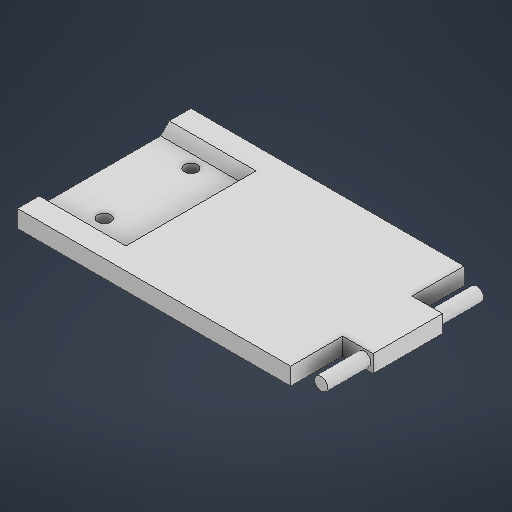
# Autodesk Inventor part: upper
Saved by Autodesk Inventor 2026.1 (Build 301233020, 233B)
## iProperties
Created: 2026-08-26
Part Number: upper
Material: Generic
Document SubType Name: Modeling
Designer: pleased
Density: 1 g/cm^3
Appearance: Default
Author: pleased
Autodesk Inventor part; units mm, degrees
ref_plane "YZ Plane" through (0, 0, 0) normal (1, 0, 0) x (0, 1, 0)
ref_plane "XZ Plane" through (0, 0, 0) normal (0, 1, 0) x (-1, 0, 0)
ref_plane "XY Plane" through (0, 0, 0) normal (0, 0, 1) x (1, 0, 0)
sketch "Sketch1" plane through (0, 0, 0) normal (0, 1, 0) x (-1, 0, 0)
  point P0 (0, 0)
sketch "Sketch2" plane through (0, 0, 0) normal (0, 1, 0) x (-1, 0, 0)
  point P0 (0, 0)
sketch "Sketch3" plane through (0, 0, 0) normal (0, 1, 0) x (-1, 0, 0)
  point P0 (0, 0)
sketch "Sketch4" plane through (0, 0, 0) normal (0, 1, 0) x (-1, 0, 0)
  line L0 (35, 20) -> (-35, 20)
  line L1 (-35, 20) -> (-35, -20)
  line L2 (-35, -20) -> (35, -20)
  line L3 (35, -20) -> (35, 20)
  line L4 (35, 20) -> (-35, -20) construction
  line L5 (-35, 20) -> (35, -20) construction
  point P0 (0, 0)
  dimension "d0" = 70
  dimension "d1" = 40
  constraints: 12 end point, 2 midpoint, 2 parallel, 1 horizontal, 1 perpendicular
  measures "d0" distance of L2.end L1.end
  measures "d1" distance of L1.end L0.end
extrude "Extrusion1" add sketch "Sketch4" along normal blind 2
sketch "Sketch5" plane through (0, 2, 0) normal (0, 1, 0) x (1, 0, 0)
  line L0 (-35, 20) -> (-35, -20) projected
  line L1 (-35, 0) -> (-25, 0)
  line L2 (-25, 0) -> (-25, 10)
  line L3 (-25, 10) -> (-25, -10)
  circle A0 centre (-25, -10) radius 1.5
  circle A1 centre (-25, 10) radius 1.5
  point P0 (0, 0)
  dimension "d4" = 10
  dimension "d5" = 10
  dimension "d6" = 20
  dimension "d7" = 3
  dimension "d8" = 3
  constraints: 6 end point, 2 centre point, 2 coincident, 1 horizontal, 1 midpoint, 1 perpendicular, 1 point on line
  measures "d4" distance of L1.start L1.end
  measures "d5" distance of L1.end L2.end
  measures "d6" distance of L2.end L3.end
  measures "d7" diameter of A0
  measures "d8" diameter of A1
extrude "Extrusion2" cut sketch "Sketch5" against normal blind 3
sketch "Sketch6" plane through (0, 2, 0) normal (0, 1, 0) x (1, 0, 0)
  line L0 (-35, -20) -> (35, -20) projected
  line L1 (35, 20) -> (-35, 20) projected
  line L2 (35, -20) -> (-15, -20)
  line L3 (-15, -20) -> (-15, 20)
  line L4 (-15, 20) -> (35, 20)
  line L5 (35, 20) -> (35, -20)
  line L6 (-35, 20) -> (-35, -20) projected
  line L7 (-15, 20) -> (-35, 20)
  line L8 (-35, 20) -> (-35, 15)
  line L9 (-35, 15) -> (-15, 15)
  line L10 (-15, 15) -> (-15, 20)
  line L11 (-35, -20) -> (-15, -20)
  line L12 (-15, -20) -> (-15, -15)
  line L13 (-15, -15) -> (-35, -15)
  line L14 (-35, -15) -> (-35, -20)
  point P0 (0, 0)
  dimension "d11" = 50
  dimension "d12" = 5
  dimension "d13" = 5
  constraints: 24 end point, 6 parallel, 3 horizontal, 3 perpendicular, 3 point on line
  measures "d11" distance of L3.end L4.end
  measures "d12" distance of L8.end L7.end
  measures "d13" distance of L12.end L11.end
extrude "Extrusion3" add sketch "Sketch6" along normal blind 2 contours L6 L13 L3 L0 | L3 L1 L5 L0 | L6 L1 L3 L9
chamfer "Chamfer1" distance 2 angle 45 3 edges at (-25, 2, 15) (-15, 2, 0) (-25, 2, -15)
sketch "Sketch7" plane through (0, 4, 0) normal (0, 1, 0) x (1, 0, 0)
  line L0 (35, -20) -> (35, 20) projected
  line L1 (35, -20) -> (28, -20)
  line L2 (28, -20) -> (28, -8)
  line L3 (28, -8) -> (35, -8)
  line L4 (35, -8) -> (35, -20)
  line L5 (35, 20) -> (28, 20)
  line L6 (28, 20) -> (28, 8)
  line L7 (28, 8) -> (35, 8)
  line L8 (35, 8) -> (35, 20)
  point P0 (0, 0)
  dimension "d19" = 7
  dimension "d20" = 12
  dimension "d21" = 12
  constraints: 16 end point, 4 parallel, 2 horizontal, 2 perpendicular, 1 point on line
  measures "d19" distance of L2.end L3.end
  measures "d20" distance of L1.end L2.end
  measures "d21" distance of L6.end L5.end
extrude "Extrusion4" cut sketch "Sketch7" against normal blind 4
sketch "Sketch8" plane through (28, 4, 8) normal (0, 0, 1) x (1, 0, 0)
  line L0 (7, -4) -> (7, 0) projected
  line L1 (7, 0) -> (3, -4)
  line L2 (0, -4) -> (7, -4) projected
  line L3 (7, 0) -> (12.6569, 0) construction
  circle A0 centre (5, -2) radius 1.5
  point P0 (-28, -4)
  dimension "d24" = 135
  dimension "d25" = 3
  constraints: 4 end point, 1 centre point, 1 equal length, 1 horizontal, 1 midpoint, 1 point on line
  measures "d24" angle of L1 L3
  measures "d25" diameter of A0
extrude "Extrusion5" add sketch "Sketch8" along normal blind 10 contours A0 L1 | L1 A0
sketch "Sketch9" plane through (35, 4, -8) normal (0, 0, -1) x (-1, 0, 0)
  circle A0 centre (2, -2) radius 1.5 projected
  circle A1 centre (2, -2) radius 1.5
  point P0 (35, -4)
  constraints: 1 centre point, 1 coincident
extrude "Extrusion6" add sketch "Sketch9" along normal blind 10
equation "\"d9\" = d7"
body "Solid1"
